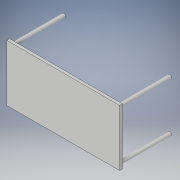
# Autodesk Inventor part: PythonKukaTable
Saved by Autodesk Inventor 2019.1 (Build 231200000, 200)
## iProperties
Created: 2020-09-13
Part Number: PythonKukaTable
Material: Generic
Document SubType Name: Modeling
Designer: lucas
Density: 1 g/cm^3
Appearance: Default
Author: lucas
Autodesk Inventor part; units mm, degrees
ref_plane "YZ Plane" through (0, 0, 0) normal (1, 0, 0) x (0, 1, 0)
ref_plane "XZ Plane" through (0, 0, 0) normal (0, 1, 0) x (-1, 0, 0)
ref_plane "XY Plane" through (0, 0, 0) normal (0, 0, 1) x (1, 0, 0)
sketch "Sketch1" plane through (0, 0, 0) normal (0, 0, 1) x (1, 0, 0)
  line L0 (-1000, 500) -> (1000, 500)
  line L1 (1000, 500) -> (1000, -500)
  line L2 (1000, -500) -> (-1000, -500)
  line L3 (-1000, -500) -> (-1000, 500)
  point P0 (0, 0)
  dimension "d0" = 2000
  dimension "d1" = 1000
  dimension "d2" = 500
  dimension "d3" = 1000
  constraints: 8 end point, 2 parallel, 1 horizontal, 1 perpendicular
  measures "d0" distance of L0.start L0.end
  measures "d1" distance of L2.end L0.start
  measures "d2" distance from line of point (0, 0) L0
  measures "d3" distance from line of point (0, 0) L3
extrude "Extrusion1" add sketch "Sketch1" along normal blind 50
sketch "Sketch2" plane through (0, 0, 0) normal (0, 0, -1) x (-1, 0, 0)
  circle A0 centre (940, 440) radius 30
  circle A1 centre (-940, 440) radius 30
  circle A2 centre (-940, -440) radius 30
  circle A3 centre (940, -440) radius 30
  line L0 (1000, 500) -> (-1000, 500) projected
  line L1 (-1000, 500) -> (-1000, -500) projected
  line L2 (1000, -500) -> (1000, 500) projected
  line L3 (-1000, -500) -> (1000, -500) projected
  point P0 (0, 0)
  dimension "d6" = 60
  dimension "d7" = 60
  dimension "d8" = 60
  dimension "d9" = 60
  dimension "d10" = 60
  dimension "d11" = 60
  dimension "d12" = 60
  dimension "d13" = 60
  dimension "d14" = 60
  dimension "d15" = 60
  dimension "d16" = 60
  dimension "d17" = 60
  constraints: 4 centre point
  measures "d6" diameter of A1
  measures "d7" distance from line of L0 A1.centre
  measures "d8" distance from line of L1 A1.centre
  measures "d9" distance from line of L0 A0.centre
  measures "d10" diameter of A0
  measures "d11" distance from line of L2 A0.centre
  measures "d12" diameter of A2
  measures "d13" distance from line of L3 A2.centre
  measures "d14" distance from line of L1 A2.centre
  measures "d15" diameter of A3
  measures "d16" distance from line of L3 A3.centre
  measures "d17" distance from line of L2 A3.centre
extrude "Extrusion2" add sketch "Sketch2" along normal blind 900 contours A0 | A1 | A2 | A3
equation "\"d1\" = 0.5 * d0"
equation "\"d2\" = 0.5 * d1"
equation "\"d3\" = 0.5 * d0"
equation "\"d7\" = d6"
equation "\"d8\" = d7"
equation "\"d9\" = d7"
equation "\"d10\" = d6"
equation "\"d11\" = d8"
equation "\"d12\" = d6"
equation "\"d13\" = d7"
equation "\"d14\" = d8"
equation "\"d15\" = d6"
equation "\"d16\" = d7"
equation "\"d17\" = d8"
body "Solid1"
